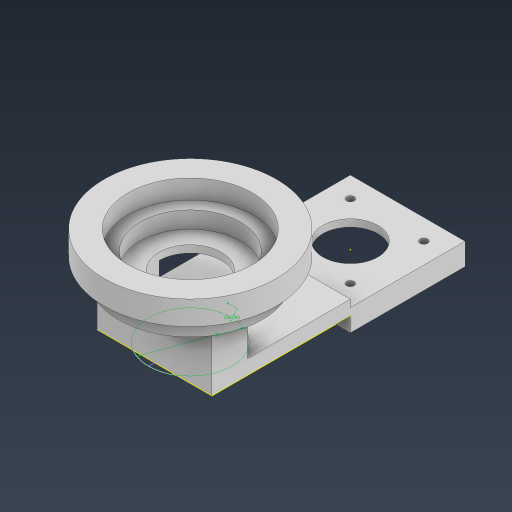
# Autodesk Inventor part: Base_top
Saved by Autodesk Inventor 2024 (Build 280153000, 153)
## iProperties
Created: 2025-10-20
Part Number: Base_top
Material: Generic
Document SubType Name: Modeling
Designer: Piter
Density: 1 g/cm^3
Appearance: Default
Author: Piter
Autodesk Inventor part; units mm, degrees
ref_plane "YZ Plane" through (0, 0, 0) normal (1, 0, 0) x (0, 1, 0)
ref_plane "XZ Plane" through (0, 0, 0) normal (0, 1, 0) x (-1, 0, 0)
ref_plane "XY Plane" through (0, 0, 0) normal (0, 0, 1) x (1, 0, 0)
sketch "Sketch1" plane through (0, 0, 0) normal (0, 1, 0) x (-1, 0, 0)
  line L0 (-21, 21) -> (21, 21)
  line L1 (21, 21) -> (21, -21)
  line L2 (21, -21) -> (-21, -21)
  line L3 (-21, -21) -> (-21, 21)
  line L4 (-21, 21) -> (21, -21) construction
  line L5 (21, 21) -> (-21, -21) construction
  line L6 (-15.3795, 15.3795) -> (15.3795, 15.3795) construction
  line L7 (15.3795, 15.3795) -> (15.3795, -15.3795) construction
  line L8 (15.3795, -15.3795) -> (-15.3795, -15.3795) construction
  line L9 (-15.3795, -15.3795) -> (-15.3795, 15.3795) construction
  line L10 (-15.3795, 15.3795) -> (15.3795, -15.3795) construction
  line L11 (15.3795, 15.3795) -> (-15.3795, -15.3795) construction
  circle A0 centre (15.3795, 15.3795) radius 1.55
  circle A1 centre (15.3795, -15.3795) radius 1.55
  circle A2 centre (-15.3795, -15.3795) radius 1.55
  circle A3 centre (-15.3795, 15.3795) radius 1.55
  circle A4 centre (0, 0) radius 11.5
  line L12 (-24, 24) -> (24, 24)
  line L13 (24, 24) -> (24, -24)
  line L14 (24, -24) -> (-24, -24)
  line L15 (-24, -24) -> (-24, 24)
  line L16 (-24, 24) -> (24, -24) construction
  line L17 (24, 24) -> (-24, -24) construction
  dimension "d0" = 42
  dimension "d1" = 42
  dimension "d2" = 30.759
  dimension "d3" = 30.759
  dimension "d4" = 3.1
  dimension "d5" = 3.1
  dimension "d6" = 3.1
  dimension "d7" = 3.1
  dimension "d8" = 23
  dimension "d11" = 3
  dimension "d12" = 3
  constraints: 36 end point, 6 midpoint, 6 parallel, 5 centre point, 5 coincident, 3 horizontal, 3 perpendicular
  measures "d0" distance of L1.end L2.end
  measures "d1" distance of L0.end L1.end
  measures "d2" distance of L7.end L8.end
  measures "d3" distance of L6.end L7.end
  measures "d4" diameter of A0
  measures "d5" diameter of A1
  measures "d6" diameter of A2
  measures "d7" diameter of A3
  measures "d8" diameter of A4
  measures "d11" distance between parallel lines of L2 L14
  measures "d12" distance between parallel lines of L1 L13
extrude "Extrusion1" add sketch "Sketch1" along normal blind 3 contours L0 L1 L2 L3
extrude "Extrusion2" add sketch "Sketch1" along normal blind 3 and the other way blind 6.2 contours L12 L13 L14 L15
sketch "Sketch2" plane through (0, 3, 0) normal (0, 1, 0) x (1, 0, 0)
  line L0 (0, 0) -> (0, -64.8507) construction
  circle A0 centre (0, -67) radius 10.5
  line L1 (24, 24) -> (-24, 24) projected
  line L2 (-24, 24) -> (-24, -24) projected
  line L3 (-24, -24) -> (24, -24) projected
  line L4 (24, -24) -> (24, 24) projected
  circle A1 centre (0, 0) radius 11.5 projected
  circle A2 centre (15.3795, -15.3795) radius 1.55 projected
  circle A3 centre (15.3795, 15.3795) radius 1.55 projected
  circle A4 centre (-15.3795, 15.3795) radius 1.55 projected
  circle A5 centre (-15.3795, -15.3795) radius 1.55 projected
  line L5 (-24, -24) -> (-24, -82)
  line L6 (-24, -82) -> (24, -82)
  line L7 (24, 24) -> (24, -24) projected
  line L8 (24, -82) -> (24, -24)
  circle A6 centre (0, -67) radius 13.05
  point P0 (0, -82)
  dimension "d17" = 21
  dimension "d18" = 67
  dimension "d19" = 15
  dimension "d20" = 26.1
  constraints: 8 end point, 2 centre point, 2 perpendicular, 2 vertical, 1 coincident, 1 midpoint, 1 point on line
  measures "d17" diameter of A0
  measures "d18" distance of L0.start A0.centre
  measures "d19" distance of point (0, -82) A0.centre
  measures "d20" diameter of A6
extrude "Extrusion3" add sketch "Sketch2" along normal blind 3 contours L8 L6 L5 L3
extrude "Extrusion4" add sketch "Sketch2" against normal blind 3 contours L8 L6 L5 L3 | A6
sketch "Sketch3" plane through (0, 6, 0) normal (0, 1, 0) x (1, 0, 0)
  line L0 (-24, -24) -> (-24, -82) projected
  line L1 (-24, -82) -> (24, -82) projected
  line L2 (24, -82) -> (24, -24) projected
  line L3 (24, -24) -> (-24, -24) projected
  circle A0 centre (0, -67) radius 13.05 projected
  circle A1 centre (0, -67) radius 10.5 projected
  line L4 (-13.05, -67) -> (-24, -67)
  line L5 (13.05, -67) -> (24, -67)
  point P0 (0, 0)
  constraints: 4 end point, 4 point on line, 2 point on circle, 1 perpendicular
extrude "Extrusion5" add sketch "Sketch3" along normal blind 20 contours L4 A0 L5 L2 L1 L0
sketch "Sketch4" plane through (0, 26, 0) normal (0, 1, 0) x (1, 0, 0)
  line L0 (24, -82) -> (24, -67) projected
  line L1 (24, -67) -> (13.05, -67) projected
  arc A0 (-13.05, -67) -> (13.05, -67) centre (0, -67) ccw projected
  line L2 (-13.05, -67) -> (-24, -67) projected
  line L3 (-24, -67) -> (-24, -82) projected
  line L4 (-24, -82) -> (24, -82) projected
  circle A1 centre (0, -67) radius 21
  circle A2 centre (0, -67) radius 26.05
  arc A3 (13.05, -67) -> (-13.05, -67) centre (0, -67) ccw projected
  point P0 (0, 0)
  point P1 (14.6969, -82)
  point P2 (21, -67)
  point P3 (24, -77.1293)
  point P4 (-24, -77.1293)
  point P5 (-21, -67)
  point P6 (-14.6969, -82)
  point P7 (-21.2979, -82)
  point P8 (21.2979, -82)
  dimension "d27" = 42
  dimension "d28" = 52.1
  constraints: 2 centre point, 2 coincident
  measures "d27" diameter of A1
  measures "d28" diameter of A2
extrude "Extrusion6" add sketch "Sketch4" along normal blind 7 contours A2 L4 A1 L1 L0 | L0 L1 A1 L2 L3 A2 | A2 L4 A1 | A2 L3 L2 A1 L4
extrude "Extrusion7" add sketch "Sketch4" against normal blind 3 contours L0 L1 A1 L2 L3 A2 | A2 L4 A1 | A1 L4 | L4 A1 L2 A0 L1 | L1 A3 L2 A1
sketch "Sketch5" plane through (0, 33, 67) normal (0, 1, 0) x (1, 0, 0)
  circle A0 centre (0, 0) radius 26.05 projected
  circle A1 centre (0, 0) radius 21 projected
  circle A2 centre (0, 0) radius 30
  point P0 (0, 67)
  dimension "d33" = 60
  constraints: 1 centre point, 1 coincident
  measures "d33" diameter of A2
extrude "Extrusion8" add sketch "Sketch5" along normal blind 8 and the other way blind 10 contours A2
sketch "Sketch6" plane through (0, 41, 67) normal (0, 1, 0) x (1, 0, 0)
  circle A0 centre (0, 0) radius 30 projected
  circle A1 centre (0, 0) radius 26.05 projected
  circle A2 centre (0, 0) radius 36
  point P0 (0, 67)
  dimension "d38" = 72
  constraints: 1 centre point, 1 coincident
  measures "d38" diameter of A2
extrude "Extrusion9" add sketch "Sketch6" against normal blind 10 contours A2
sketch "Sketch7" plane through (0, 0, 0) normal (0, -1, 0) x (1, 0, 0)
  line L0 (13.05, 67) -> (24, 67) projected
  line L1 (-24, 82) -> (-24, 24) projected
  line L2 (24, 24) -> (-24, 24) projected
  line L3 (24, 24) -> (24, 82) projected
  line L4 (24, 82) -> (-24, 82) projected
  circle A0 centre (0, 67) radius 10.5 projected
  circle A1 centre (0, 67) radius 17.5
  line L5 (0, 84.5) -> (0, 49.5)
  circle A2 centre (0, 49.5) radius 2
  circle A3 centre (15.1554, 75.75) radius 2
  circle A4 centre (-15.1554, 75.75) radius 2
  point P0 (0, 0)
  dimension "d41" = 35
  dimension "d43" = 4
  dimension "d46" = 360
  constraints: 4 centre point, 3 point on circle, 2 end point, 1 coincident, 1 vertical, 7 other
  measures "d41" diameter of A1
  measures "d43" diameter of A2
body "Solid1"
